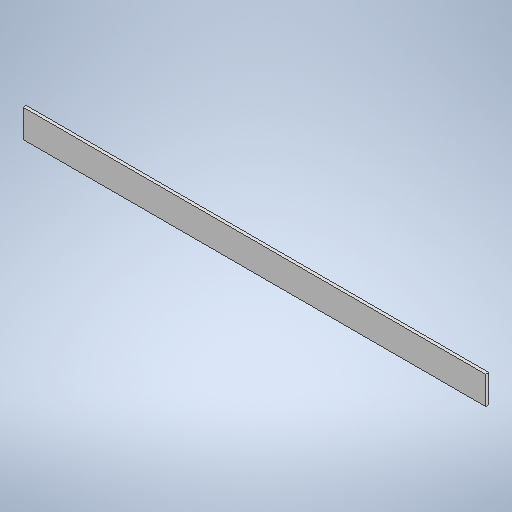
# Autodesk Inventor part: back support
Saved by Autodesk Inventor 2025.4 (Build 294407000, 407)
## iProperties
Created: 2026-05-23
Part Number: back support
Material: Generic
Document SubType Name: Modeling
Designer: lenovo
Density: 1 g/cm^3
Appearance: Default
Author: lenovo
Autodesk Inventor part; units mm, degrees
ref_plane "YZ Plane" through (0, 0, 0) normal (1, 0, 0) x (0, 1, 0)
ref_plane "XZ Plane" through (0, 0, 0) normal (0, 1, 0) x (-1, 0, 0)
ref_plane "XY Plane" through (0, 0, 0) normal (0, 0, 1) x (1, 0, 0)
sketch "Sketch1" plane through (0, 0, 0) normal (0, 0, 1) x (1, 0, 0)
  line L0 (-219.5, -13.25) -> (219.5, -13.25)
  line L1 (219.5, -13.25) -> (219.5, 13.25)
  line L2 (219.5, 13.25) -> (-219.5, 13.25)
  line L3 (-219.5, 13.25) -> (-219.5, -13.25)
  line L4 (-219.5, -13.25) -> (219.5, 13.25) construction
  line L5 (219.5, -13.25) -> (-219.5, 13.25) construction
  point P0 (0, 0)
  dimension "d0" = 26.5
  dimension "d1" = 439
  constraints: 12 end point, 2 midpoint, 2 parallel, 1 horizontal, 1 perpendicular
  measures "d0" distance of L1.end L0.end
  measures "d1" distance of L1.end L2.end
extrude "Extrusion1" add sketch "Sketch1" along normal blind 3
body "Solid1"
